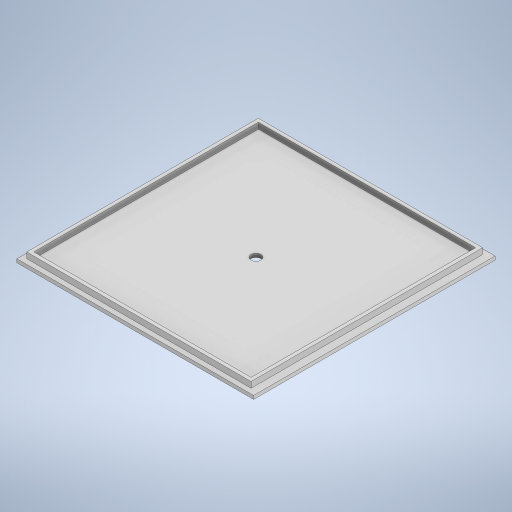
# Autodesk Inventor part: TAPA GENERAL
Saved by Autodesk Inventor 2024 (Build 280153000, 153)
## iProperties
Created: 2024-05-27
Part Number: TAPA GENERAL
Material: Generic
Document SubType Name: Modeling
Designer: samue
Density: 1 g/cm^3
Appearance: Default
Author: samue
## iProperties of the stored document TAPA GENERAL_3DPrint.ipt
Created: 2024-05-27
Part Number: TAPA GENERAL_3DPrint
Material: Generic
Document SubType Name: Modeling
Designer: samue
Density: 1 g/cm^3
Appearance: Default
Author: samue
Autodesk Inventor part; units mm, degrees
ref_plane "YZ Plane" through (0, 0, 0) normal (1, 0, 0) x (0, 1, 0)
ref_plane "XZ Plane" through (0, 0, 0) normal (0, 1, 0) x (-1, 0, 0)
ref_plane "XY Plane" through (0, 0, 0) normal (0, 0, 1) x (1, 0, 0)
sketch "Sketch1" plane through (0, 0, 0) normal (0, 1, 0) x (-1, 0, 0)
  line L0 (50.5, 51.5) -> (-50.5, 51.5)
  line L1 (-50.5, 51.5) -> (-50.5, -51.5)
  line L2 (-50.5, -51.5) -> (50.5, -51.5)
  line L3 (50.5, -51.5) -> (50.5, 51.5)
  line L4 (50.5, 51.5) -> (-50.5, -51.5) construction
  line L5 (-50.5, 51.5) -> (50.5, -51.5) construction
  line L6 (48.4022, -49.4) -> (-47.3, -49.4)
  line L7 (-47.3, 49.4022) -> (48.4022, 49.4022)
  line L8 (48.4022, 49.4022) -> (48.4022, -49.4)
  line L9 (-47.3, -47.9892) -> (-47.3, 42.6215)
  line L10 (-47.3, -47.9892) -> (-47.3, -49.4)
  line L11 (-47.3, 42.6215) -> (-47.3, 49.4022)
  line L12 (46.9022, -47.9) -> (-45.8, -47.9)
  line L13 (-45.8, -47.9) -> (-45.8, 42.6215)
  line L14 (-45.8, 42.6215) -> (-45.8, 47.9022)
  line L15 (-45.8, 47.9022) -> (46.9022, 47.9022)
  line L16 (46.9022, 47.9022) -> (46.9022, -47.9)
  point P0 (0, 0)
  dimension "d0" = 101
  dimension "d1" = 103
  dimension "d2" = 2.1
  dimension "d3" = 3.2
  dimension "d4" = 1.5
  constraints: 34 end point, 4 parallel, 2 midpoint, 2 perpendicular, 2 vertical, 1 horizontal, 4 other
  measures "d0" distance of L2.end L1.end
  measures "d1" distance of L1.end L0.end
  measures "d2" distance between parallel lines of L2 L6
  measures "d3" distance between parallel lines of L1 L9
  measures "d4" distance between parallel lines of L8 L16
extrude "Extrusion1" add sketch "Sketch1" along normal blind 1.5 contours L3 L2 L1 L0 | L6 L10 L9 L11 L7 L8 | L12 L13 L14 L15 L16
extrude "Extrusion2" add sketch "Sketch1" along normal blind 4 contours L6 L10 L9 L11 L7 L8
sketch "Sketch2" plane through (0, 1.5, 0) normal (0, 1, 0) x (1, 0, 0)
  circle A0 centre (0, 0) radius 2.1
  dimension "d9" = 4.2
  constraints: 1 centre point, 1 coincident
  measures "d9" diameter of A0
extrude "Extrusion3" cut sketch "Sketch2" against normal blind 4
body "Solid1"
